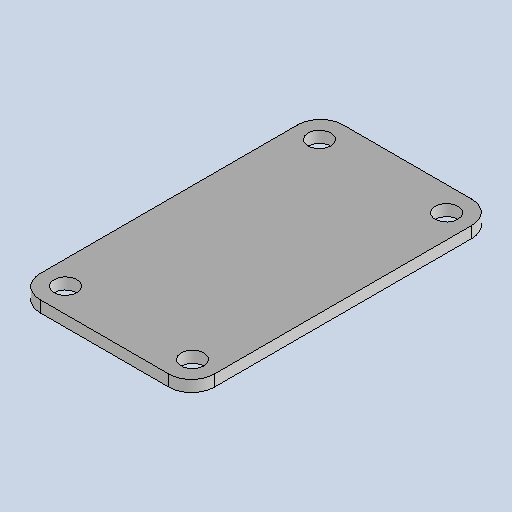
# Autodesk Inventor part: ANP 1434 BOTTOM FDS support flange
Saved by Autodesk Inventor 2025 (Build 290162010, 162A)
## iProperties
Created: 2025-06-24
Part Number: ANP 1434 BOTTOM FDS support flange
Material: Stainless Steel
Document SubType Name: Sheet Metal
Designer: admin
Mass: 103.446 g
Surface Area: 101.897 cm^2
Volume: 12.9307 cm^3
Density: 8 g/cm^3
Flat Pattern Width: 4.6 cm
Flat Pattern Length: 8 cm
Flat Pattern Area: 36.8 cm^2
Sheet Metal Rule: AISI304 2mm Die16
Sheet Metal Width: 46,000 mm
Sheet Metal Length: 80,000 mm
Sheet Metal Area: 3680,000 mm^2
Appearance: Default
Author: user
Autodesk Inventor part; units mm, degrees
ref_plane "YZ Plane" through (0, 0, 0) normal (1, 0, 0) x (0, 1, 0)
ref_plane "XZ Plane" through (0, 0, 0) normal (0, 1, 0) x (-1, 0, 0)
ref_plane "XY Plane" through (0, 0, 0) normal (0, 0, 1) x (1, 0, 0)
sketch "Sketch1" plane through (0, 0, 0) normal (0, 0, 1) x (1, 0, 0)
  line L0 (-23, -40) -> (23, -40)
  line L1 (23, -40) -> (23, 40)
  line L2 (23, 40) -> (-23, 40)
  line L3 (-23, 40) -> (-23, -40)
  line L4 (-23, -40) -> (23, 40) construction
  line L5 (23, -40) -> (-23, 40) construction
  line L6 (10, -20) -> (-10, -20)
  line L7 (-10, -20) -> (-10, 20)
  line L8 (-10, 20) -> (10, 20)
  line L9 (10, 20) -> (10, -20)
  line L10 (10, -20) -> (-10, 20) construction
  line L11 (-10, -20) -> (10, 20) construction
  point P0 (0, 0)
  dimension "d154" = 46
  dimension "d155" = 80
  dimension "d172" = 20
  dimension "d181" = 40
  measures "d154" distance of L1.end L2.end
  measures "d155" distance of L0.end L1.end
  measures "d172" distance of L7.end L8.end
  measures "d181" distance of L6.end L7.end
extrude "Plate5" add sketch "Sketch1" along normal blind 3 contours L3 L2 L1 L0 | L6 L7 L8 L9
sketch "Sketch9" plane through (0, 0, 3) normal (0, 0, 1) x (1, 0, 0)
  circle A0 centre (16.7705, -33.541) radius 3
  line L0 (16.7705, 33.541) -> (-16.7705, 33.541) construction
  line L1 (-16.7705, 33.541) -> (-16.7705, -33.541) construction
  line L2 (-16.7705, -33.541) -> (16.7705, -33.541) construction
  line L3 (16.7705, -33.541) -> (16.7705, 33.541) construction
  line L4 (16.7705, 33.541) -> (-16.7705, -33.541) construction
  line L5 (-16.7705, 33.541) -> (16.7705, -33.541) construction
  circle A1 centre (-16.7705, -33.541) radius 3
  circle A2 centre (16.7705, 33.541) radius 3
  circle A3 centre (-16.7705, 33.541) radius 3
  circle A4 centre (0, 0) radius 37.5 construction
  line L6 (23, -40) -> (-23, -40) construction
  line L7 (23, 40) -> (23, -40) construction
  line L8 (-23, 40) -> (23, 40) construction
  line L9 (-23, -40) -> (-23, 40) construction
  circle A5 centre (0, 0) radius 22.3607 construction
  line L10 (10, 20) -> (-10, -20) construction
  dimension "d180" = 75
  dimension "d182" = 15.1393
  dimension "d174" = 6
  dimension "d183" = 33.541
  constraints: 14 end point, 9 coincident, 4 centre point, 3 equal radius, 2 midpoint, 2 parallel, 1 collinear, 1 horizontal, 1 perpendicular, 6 other
  measures "d174" diameter of A0
  measures "d183" distance of L0.start L0.end
extrude "Cut2" cut sketch "Sketch9" against normal blind 3
fillet "Corner Round1" radius 6 4 edges at (23, 40, 1.5) (-23, 40, 1.5) (-23, -40, 1.5) (23, -40, 1.5)
feature "Corner Round2" [suppressed]
body "Solid3"
